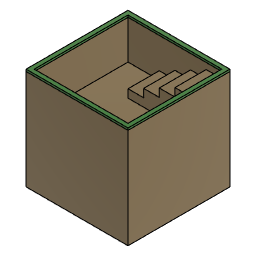
Channel first level v3 (Autodesk Fusion 360 design; units mm, degrees)
Autodesk Fusion 360 part; units mm, degrees
sketch "Skizze1" plane through (0, 0, 0) normal (0, 0, 1) x (1, 0, 0)
  line L0 (-25, 25) -> (25, 25)
  line L1 (25, 25) -> (25, -25)
  line L2 (25, -25) -> (-25, -25)
  line L3 (-25, -25) -> (-25, 25)
  line L4 (-23, 23) -> (23, 23)
  line L5 (23, 23) -> (23, -23)
  line L6 (23, -23) -> (-23, -23)
  line L7 (-23, -23) -> (-23, 23)
  line L8 (23, 23) -> (15.3333, 23)
  line L9 (15.3333, 23) -> (15.3333, 7.6667)
  line L10 (15.3333, 7.6667) -> (23, 7.6667)
  line L11 (23, 7.6667) -> (23, 23)
  line L12 (15.3333, 23) -> (7.6667, 23)
  line L13 (7.6667, 23) -> (7.6667, 7.6667)
  line L14 (7.6667, 7.6667) -> (15.3333, 7.6667)
  line L15 (15.3333, 7.6667) -> (15.3333, 23)
  line L16 (23, 7.6667) -> (-23, 7.6667) construction
  line L17 (7.6667, 23) -> (0, 23)
  line L18 (0, 23) -> (0, 7.6667)
  line L19 (0, 7.6667) -> (7.6667, 7.6667)
  line L20 (7.6667, 7.6667) -> (7.6667, 23)
  line L21 (0, 23) -> (-7.6667, 23)
  line L22 (-7.6667, 23) -> (-7.6667, 7.6667)
  line L23 (-7.6667, 7.6667) -> (0, 7.6667)
  line L24 (0, 7.6667) -> (0, 23)
  line L25 (-7.6667, 23) -> (-15.5981, 23)
  line L26 (-7.6667, 8) -> (-7.6667, 23)
  line L27 (-7.6667, 7.6667) -> (-23, 7.6667)
  line L28 (-23, 7.6667) -> (-23, 23)
  line L29 (-23, 23) -> (-7.6667, 23)
  line L30 (-7.6667, 23) -> (-7.6667, 7.6667)
  line L31 (0, 25) -> (0, -25) construction
  line L32 (-25, 0) -> (25, 0) construction
  line L33 (-7.6667, 7.6667) -> (-7.6667, -23) construction
  line L34 (-23, 7.6667) -> (-7.6667, 7.6667)
  line L35 (-7.6667, 7.6667) -> (-7.6667, 0)
  line L36 (-7.6667, 0) -> (-23, 0)
  line L37 (-23, 0) -> (-23, 7.6667)
  line L38 (-23, 0) -> (-7.6667, 0)
  line L39 (-7.6667, 0) -> (-7.6667, -7.6667)
  line L40 (-7.6667, -7.6667) -> (-23, -7.6667)
  line L41 (-23, -7.6667) -> (-23, 0)
  line L42 (-23, -7.6667) -> (-7.6667, -7.6667)
  line L43 (-7.6667, -7.6667) -> (-7.6667, -23)
  line L44 (-7.6667, -23) -> (-23, -23)
  line L45 (-23, -23) -> (-23, -7.6667)
  line L46 (-7.6667, -23) -> (0, -23)
  line L47 (0, -23) -> (0, -7.6667)
  line L48 (0, -7.6667) -> (-7.6667, -7.6667)
  line L49 (-7.6667, -7.6667) -> (-7.6667, -23)
  line L50 (0, -23) -> (7.6667, -23)
  line L51 (7.6667, -23) -> (7.6667, -7.6667)
  line L52 (7.6667, -7.6667) -> (0, -7.6667)
  line L53 (0, -7.6667) -> (0, -23)
  line L54 (7.6667, -23) -> (15.3333, -23)
  line L55 (15.3333, -23) -> (15.3333, -7.6667)
  line L56 (15.3333, -7.6667) -> (7.6667, -7.6667)
  line L57 (7.6667, -7.6667) -> (7.6667, -23)
  line L58 (-7.6667, -7.6667) -> (23, -7.6667) construction
  dimension "d1" = 2
  dimension "d2" = 7.6667
  dimension "d3" = 15.3333
  dimension "d4" = 7.6667
  dimension "d5" = 7.6667
  dimension "d6" = 7.6667
  dimension "d7" = 50
  dimension "d8" = 50
  dimension "d9" = 7.6667
  dimension "d10" = 7.6667
  dimension "d11" = 7.6667
  dimension "d12" = 7.6667
  dimension "d13" = 7.6667
  constraint horizontal L0
  constraint vertical L1
  constraint horizontal L2
  constraint vertical L3
  constraint horizontal L8
  constraint vertical L9
  constraint horizontal L10
  constraint vertical L11
  constraint horizontal L12
  constraint vertical L13
  constraint horizontal L14
  constraint vertical L15
  constraint coincident L7 L16.end
  constraint perpendicular L7 L16
  constraint horizontal L17
  constraint vertical L18
  constraint horizontal L19
  constraint vertical L20
  constraint coincident L16 L18.end
  constraint horizontal L21
  constraint vertical L22
  constraint horizontal L23
  constraint vertical L24
  constraint coincident L16 L22.end
  constraint horizontal L25
  constraint vertical L26
  constraint horizontal L27
  constraint vertical L28
  constraint horizontal L29
  constraint vertical L30
  constraint midpoint L0 L31.start
  constraint midpoint L2 L31.end
  constraint midpoint L3 L32.start
  constraint midpoint L1 L32.end
  constraint coincident origin L31
  constraint coincident origin L32
  constraint collinear L14 L16
  constraint coincident L6 L33.end
  constraint perpendicular L6 L33
  constraint horizontal L34
  constraint vertical L35
  constraint horizontal L36
  constraint vertical L37
  constraint coincident L33 L35.end
  constraint horizontal L38
  constraint vertical L39
  constraint horizontal L40
  constraint vertical L41
  constraint horizontal L42
  constraint vertical L43
  constraint horizontal L44
  constraint vertical L45
  constraint horizontal L46
  constraint vertical L47
  constraint horizontal L48
  constraint vertical L49
  constraint horizontal L50
  constraint vertical L51
  constraint horizontal L52
  constraint vertical L53
  constraint horizontal L54
  constraint vertical L55
  constraint horizontal L56
  constraint vertical L57
  constraint coincident L5 L58.end
  constraint perpendicular L5 L58
  constraint collinear L33 L39
  constraint collinear L48 L58
  constraint collinear L52 L58
  constraint collinear L56 L58
  measures "d2" distance of L9.end L10.end
  measures "d3" distance of L8.end L9.end
  measures "d4" distance of L13.end L9.end
  measures "d5" distance of L18 L20
  measures "d6" distance of L24 L26
  measures "d7" distance of L0.start L0.end
  measures "d8" distance of L0.start L2.end
  measures "d9" distance of L16 L36
  measures "d10" distance of L36 L40
  measures "d11" distance of L33 L47
  measures "d12" distance of L31 L51
  measures "d13" distance of L55 L57
extrude "Extrusion1" add sketch "Skizze1" against normal blind 50 contours L0 L1 L2 L3 | L4 L7 L22 L25 L26 L27 L28 L29 L30 L34 | L7 L27 L34 L35 L36 L37 L38 | L4 L18 L21 L22 L23 L24 L26 L30 | L7 L36 L38 L39 L40 L41 L42 | L5 L6 L10 L14 L19 L23 L35 L39 L48 L52 L55 L56 | L4 L13 L17 L18 L19 L20 L24 | L6 L7 L40 L42 L43 L44 L45 L49 | L4 L9 L12 L13 L14 L15 L20 | L6 L43 L46 L47 L48 L49 L53 | L4 L5 L8 L9 L10 L11 L15 | L6 L47 L50 L51 L52 L53 L57 | L6 L51 L54 L55 L56 L57 makes body 1 in component "Quader"
extrude "Extrusion2" cut sketch "Skizze1" against normal blind 4 contours L4 L5 L8 L9 L10 L11 L15 bodies 1 in component "Quader"
extrude "Extrusion3" cut sketch "Skizze1" against normal blind 8 contours L4 L9 L12 L13 L14 L15 L20 bodies 1 in component "Quader"
extrude "Extrusion4" cut sketch "Skizze1" against normal blind 12 contours L4 L13 L17 L18 L19 L20 L24 bodies 1 in component "Quader"
extrude "Extrusion5" cut sketch "Skizze1" against normal blind 16 contours L4 L18 L21 L22 L23 L24 L26 L30 bodies 1 in component "Quader"
extrude "Extrusion6" cut sketch "Skizze1" against normal blind 20 contours L4 L7 L22 L25 L26 L27 L28 L29 L30 L34 | L7 L27 L34 L35 L36 L37 L38 | L7 L36 L38 L39 L40 L41 L42 | L5 L6 L10 L14 L19 L23 L35 L39 L48 L52 L55 L56 | L6 L7 L40 L42 L43 L44 L45 L49 | L6 L43 L46 L47 L48 L49 L53 | L6 L47 L50 L51 L52 L53 L57 | L6 L51 L54 L55 L56 L57 bodies 1 in component "Quader"
ref_plane "Arbeitsebene1" through (0, 0, -1) normal (0, 0, 1) x (1, 0, 0)
split "Teilen1" by plane through (0, 0, -1) normal (0, 0, 1) bodies 1 makes body 2 at (-24.3333, 7.6667, 0) in component "Quader"
component "Quader" placed x (1, 0, 0) y (0, 1, 0) z (0, 0, 1) at (0, 0, 0)
equation "d2 = ( d7 - 2 * d1 ) / 6"
equation "d3 = d2 * 2"
equation "d4 = d2"
equation "d5 = d2"
equation "d6 = d2"
equation "d8 = d7"
equation "d9 = d2"
equation "d10 = d2"
equation "d11 = d2"
equation "d12 = d2"
equation "d13 = d2"
equation "h_step = 4 mm" comment "hight of one step"
equation "d17 = -h_step"
equation "d19 = -h_step * 2"
equation "d21 = 3 * -h_step"
equation "d23 = 4 * -h_step"
equation "d25 = 5 * -h_step"
